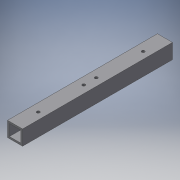
# Autodesk Inventor part: base mount
Saved by Autodesk Inventor 2018 (Build 220112000, 112)
## iProperties
Created: 2019-02-24
Part Number: base mount
Material: Generic
Document SubType Name: Modeling
Designer: s-2513225
Density: 1 g/cm^3
Appearance: Default
Author: s-2513225
Autodesk Inventor part; units mm, degrees
ref_plane "YZ Plane" through (0, 0, 0) normal (1, 0, 0) x (0, 1, 0)
ref_plane "XZ Plane" through (0, 0, 0) normal (0, 1, 0) x (-1, 0, 0)
ref_plane "XY Plane" through (0, 0, 0) normal (0, 0, 1) x (1, 0, 0)
sketch "Sketch1" plane through (0, 0, 0) normal (0, 0, 1) x (1, 0, 0)
  line L0 (0, 0) -> (25.4, 0)
  line L1 (25.4, 0) -> (25.4, 25.4)
  line L2 (25.4, 25.4) -> (0, 25.4)
  line L3 (0, 25.4) -> (0, 0)
  line L4 (3.175, 22.225) -> (22.225, 22.225)
  line L5 (22.225, 22.225) -> (22.225, 3.175)
  line L6 (22.225, 3.175) -> (3.175, 3.175)
  line L7 (3.175, 3.175) -> (3.175, 22.225)
  dimension "d0" = 25.4
  dimension "d1" = 25.4
  dimension "d2" = 3.175
  constraints: 16 end point, 4 parallel, 2 perpendicular, 1 horizontal, 3 other
  measures "d0" distance of L2.end L1.end
  measures "d1" distance of L1.end L0.end
  measures "d2" distance between parallel lines of L2 L4
extrude "Extrusion1" add sketch "Sketch1" along normal blind 190.5 and the other way blind 12.7
sketch "Sketch2" plane through (0, 25.4, -12.7) normal (0, 1, 0) x (1, 0, 0)
  line L0 (13.8579, 0) -> (13.8579, -12.7) construction
  line L1 (13.8579, -203.2028) -> (13.8579, -190.5028) construction
  circle A0 centre (13.8579, -190.5028) radius 2.5797
  circle A1 centre (13.8579, -12.7) radius 2.5797
  point P0 (0, -12.7)
  dimension "d6" = 12.7
  dimension "d7" = 12.7
  dimension "d8" = 5.1594
  dimension "d9" = 5.1594
  constraints: 4 end point, 2 centre point, 2 coincident, 2 vertical
  measures "d6" distance of L0.start L0.end
  measures "d7" distance of L1.start L1.end
  measures "d8" diameter of A0
  measures "d9" diameter of A1
extrude "Extrusion2" cut sketch "Sketch2" against normal blind 152.4
sketch "Sketch3" plane through (0, 0, 190.5) normal (0, 0, 1) x (1, 0, 0)
  line L0 (3.175, 3.175) -> (3.175, 22.225) projected
  line L1 (22.225, 22.225) -> (22.225, 3.175) projected
  line L2 (22.225, 3.175) -> (3.175, 3.175) projected
  line L3 (3.175, 3.175) -> (3.175, 22.225) projected
  line L4 (3.175, 22.225) -> (22.225, 22.225) projected
  line L5 (0, 0) -> (25.4, 0) projected
  line L6 (25.4, 0) -> (25.4, 25.4) projected
  line L7 (25.4, 25.4) -> (0, 25.4) projected
  line L8 (0, 25.4) -> (0, 0) projected
extrude "Extrusion3" add sketch "Sketch3" along normal blind 25.4
sketch "Sketch4" plane through (0, 0, -12.7) normal (0, 0, -1) x (-1, 0, 0)
  line L0 (-22.225, 3.175) -> (-22.225, 22.225) projected
  line L1 (-22.225, 22.225) -> (-3.175, 22.225) projected
  line L2 (-3.175, 22.225) -> (-3.175, 3.175) projected
  line L3 (-3.175, 3.175) -> (-22.225, 3.175) projected
  line L4 (-25.4, 0) -> (0, 0) projected
  line L5 (0, 0) -> (0, 25.4) projected
  line L6 (0, 25.4) -> (-25.4, 25.4) projected
  line L7 (-25.4, 25.4) -> (-25.4, 0) projected
extrude "Extrusion4" add sketch "Sketch4" along normal blind 25.4
sketch "Sketch5" plane through (0, 25.4, 215.9) normal (0, 1, 0) x (1, 0, 0)
  line L0 (3.175, 0) -> (22.225, 0) construction
  line L1 (12.7, 0) -> (12.7, 116.459) construction
  line L2 (22.225, 254) -> (3.175, 254) construction
  line L3 (12.7, 254) -> (12.7, 137.541) construction
  circle A0 centre (12.7, 137.541) radius 2.5797
  circle A1 centre (12.7, 116.459) radius 2.5797
  point P0 (0, 215.9)
  dimension "d18" = 116.459
  dimension "d19" = 116.459
  dimension "d20" = 5.1594
  dimension "d21" = 5.1594
  constraints: 4 end point, 2 centre point, 2 coincident, 2 midpoint, 2 vertical
  measures "d18" distance of L1.start L1.end
  measures "d19" distance of L3.start L3.end
  measures "d20" diameter of A0
  measures "d21" diameter of A1
extrude "Extrusion5" cut sketch "Sketch5" against normal blind 50.8
body "Solid1"
